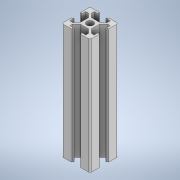
# Autodesk Inventor part: ITEM_Profil
Saved by Autodesk Inventor 2021 (Build 250183000, 183)
## iProperties
Created: 2023-11-23
Part Number: ITEM_Profil
Material: Generisch
Document SubType Name: Modeling
Designer: install
Density: 1 g/cm^3
Appearance: Vorgabe
Author: install
Autodesk Inventor part; units mm, degrees
ref_plane "YZ Plane" through (0, 0, 0) normal (1, 0, 0) x (0, 1, 0)
ref_plane "XZ Plane" through (0, 0, 0) normal (0, 1, 0) x (-1, 0, 0)
ref_plane "XY Plane" through (0, 0, 0) normal (0, 0, 1) x (1, 0, 0)
sketch "Skizze2" plane through (0, 0, 0) normal (0, 1, 0) x (-1, 0, 0)
  line L0 (0, 0) -> (30, 0)
  line L1 (30, 0) -> (30, 30)
  line L2 (30, 30) -> (0, 30)
  line L3 (0, 30) -> (0, 0)
  line L4 (28, 28) -> (2, 28)
  line L5 (2, 28) -> (2, 2)
  line L6 (2, 2) -> (28, 2)
  line L7 (28, 2) -> (28, 28)
  line L8 (19, 30) -> (19, 28)
  line L9 (11, 30) -> (11, 28)
  line L10 (23.5, 28) -> (23.5, 25)
  line L11 (19.5, 21) -> (10.5, 21)
  line L12 (6.5, 25) -> (6.5, 28)
  line L13 (23.5, 25) -> (19.5, 21)
  line L14 (6.5, 25) -> (10.5, 21)
  line L15 (5, 6.5) -> (2, 6.5)
  line L16 (9, 19.5) -> (9, 10.5)
  line L17 (5, 23.5) -> (9, 19.5)
  line L18 (2, 23.5) -> (5, 23.5)
  line L19 (0, 19) -> (2, 19)
  line L20 (0, 11) -> (2, 11)
  line L21 (5, 6.5) -> (9, 10.5)
  line L22 (23.5, 5) -> (23.5, 2)
  line L23 (10.5, 9) -> (19.5, 9)
  line L24 (6.5, 5) -> (10.5, 9)
  line L25 (6.5, 2) -> (6.5, 5)
  line L26 (11, 0) -> (11, 2)
  line L27 (19, 0) -> (19, 2)
  line L28 (23.5, 5) -> (19.5, 9)
  line L29 (25, 23.5) -> (28, 23.5)
  line L30 (21, 10.5) -> (21, 19.5)
  line L31 (25, 6.5) -> (21, 10.5)
  line L32 (28, 6.5) -> (25, 6.5)
  line L33 (30, 11) -> (28, 11)
  line L34 (30, 19) -> (28, 19)
  line L35 (25, 23.5) -> (21, 19.5)
  circle A0 centre (15, 15) radius 3.5
  line L36 (20, 30) -> (20, 29)
  line L37 (20, 29) -> (19, 29)
  line L38 (11, 29) -> (10, 29)
  line L39 (10, 29) -> (10, 30)
  line L40 (1, 10) -> (0, 10)
  line L41 (1, 11) -> (1, 10)
  line L42 (1, 20) -> (1, 19)
  line L43 (0, 20) -> (1, 20)
  line L44 (20, 1) -> (20, 0)
  line L45 (19, 1) -> (20, 1)
  line L46 (10, 1) -> (11, 1)
  line L47 (10, 0) -> (10, 1)
  line L48 (29, 20) -> (30, 20)
  line L49 (29, 19) -> (29, 20)
  line L50 (29, 10) -> (29, 11)
  line L51 (30, 10) -> (29, 10)
  point P0 (23.5, 21)
  point P1 (6.5, 21)
  point P2 (9, 6.5)
  point P3 (9, 23.5)
  point P4 (23.5, 9)
  point P5 (6.5, 9)
  point P6 (21, 23.5)
  point P7 (21, 6.5)
  dimension "d23" = 30
  dimension "d24" = 30
  dimension "d25" = 2
  dimension "d26" = 2
  dimension "d27" = 2
  dimension "d28" = 2
  dimension "d29" = 8
  dimension "d30" = 11
  dimension "d32" = 6.5
  dimension "d33" = 17
  dimension "d34" = 9
  dimension "d35" = 4
  dimension "d36" = 4
  dimension "d37" = 4
  dimension "d38" = 4
  dimension "d39" = 15
  dimension "d40" = 15
  dimension "d43" = 360
  dimension "d45" = 7
  dimension "d46" = 1
  dimension "d47" = 1
  dimension "d48" = 1
  dimension "d49" = 1
  dimension "d52" = 360
  constraints: 104 end point, 24 point on line, 8 perpendicular, 4 parallel, 3 horizontal, 2 midpoint, 2 vertical, 1 centre point, 1 coincident, 118 other
  measures "d23" distance between parallel lines of L3 L1
  measures "d24" distance between parallel lines of L0 L2
  measures "d25" distance between parallel lines of L2 L4
  measures "d26" distance between parallel lines of L1 L7
  measures "d27" distance between parallel lines of L0 L6
  measures "d28" distance between parallel lines of L3 L5
  measures "d29" distance between parallel lines of L9 L8
  measures "d30" distance between parallel lines of L3 L9
  measures "d32" distance between parallel lines of L3 L12
  measures "d33" distance between parallel lines of L12 L10
  measures "d34" distance between parallel lines of L2 L11
  measures "d35" distance of L10.end point (23.5, 21)
  measures "d36" distance of L11.start point (23.5, 21)
  measures "d37" distance of L12.start point (6.5, 21)
  measures "d38" distance of L11.end point (6.5, 21)
  measures "d39" distance from line of L0 point (15, 15)
  measures "d40" distance from line of L3 point (15, 15)
  measures "d45" diameter of A0
  measures "d46" distance between parallel lines of L2 L37
  measures "d47" distance between parallel lines of L8 L36
  measures "d48" distance between parallel lines of L2 L38
  measures "d49" distance between parallel lines of L9 L39
extrude "Extrusion1" add sketch "Skizze2" along normal blind 123 contours L3 L40 L41 L20 L5 L6 L26 L46 L47 L0 | L44 L45 L27 L6 L7 L33 L50 L51 L1 L0 | L3 L2 L39 L38 L9 L4 L5 L19 L42 L43 | L6 L5 L15 L21 L16 L17 L18 L4 L12 L14 L11 L13 L10 L7 L29 L35 L30 L31 L32 L22 L28 L23 L24 L25 | L48 L49 L34 L7 L4 L8 L37 L36 L2 L1
fillet "Rundung1" radius 2 4 edges at (0, 61.5, 30) (0, 61.5, 0) (-30, 61.5, 0) (-30, 61.5, 30)
